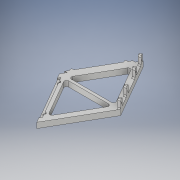
# Autodesk Inventor part: Hex_Servo_Base
Saved by Autodesk Inventor 2019 (Build 230136000, 136)
## iProperties
Created: 2019-09-23
Part Number: Hex_Servo_Base
Material: Generic
Document SubType Name: Modeling
Designer: Jorian Brusind
Density: 1 g/cm^3
Appearance: Default
Author: Jorian Brusind
Autodesk Inventor part; units mm, degrees
ref_plane "YZ Plane" through (0, 0, 0) normal (1, 0, 0) x (0, 1, 0)
ref_plane "XZ Plane" through (0, 0, 0) normal (0, 1, 0) x (-1, 0, 0)
ref_plane "XY Plane" through (0, 0, 0) normal (0, 0, 1) x (1, 0, 0)
sketch "Sketch5" plane through (0, 0, 0) normal (0, 1, 0) x (-1, 0, 0)
  line L0 (0, 0) -> (-90, 0)
  line L1 (-90, 0) -> (-45, 77.9423)
  line L2 (-90, 0) -> (-45, -77.9423)
  line L3 (-90, 0) -> (0, 0) construction
  line L4 (-45, 77.9423) -> (0, 0)
  line L5 (-45, -77.9423) -> (0, 0)
  line L6 (11.547, 0) -> (-45, 97.9423)
  line L7 (-45, 97.9423) -> (-101.547, 0)
  line L8 (-101.547, 0) -> (-45, -97.9423)
  line L9 (-45, -97.9423) -> (11.547, 0)
  line L10 (-90, -2.5) -> (0, -2.5)
  line L11 (0, -2.5) -> (0, 2.5)
  line L12 (0, 2.5) -> (-90, 2.5)
  line L13 (-90, 2.5) -> (-90, -2.5)
  line L14 (-90, -2.5) -> (0, 2.5) construction
  line L15 (0, -2.5) -> (-90, 2.5) construction
  point P0 (-45, 0)
  dimension "d32" = 90
  dimension "d33" = 90
  dimension "d34" = 60
  dimension "d35" = 90
  dimension "d36" = 60
  dimension "d37" = 60
  dimension "d38" = 10
  dimension "d39" = 5
  constraints: 32 end point, 3 midpoint, 3 parallel, 2 horizontal, 1 equal length, 1 perpendicular, 3 other
  measures "d32" distance of L0.start L0.end
  measures "d33" distance of L0.end L1.end
  measures "d34" angle of L0 L1
  measures "d35" distance of L0.end L2.end
  measures "d36" angle of L2 L3
  measures "d37" angle of L2 L5
  measures "d38" distance between parallel lines of L4 L6
  measures "d39" distance of L11.end L10.end
extrude "Extrusion4" add sketch "Sketch5" along normal blind 10 contours L5 L10 L2 L0 | L0 L1 L12 L4 | L11 L10 L5 | L4 L12 L11 | L13 L12 L1 | L2 L10 L13 | L9 L8 L7 L6
sketch "Sketch6" plane through (0, 10, 0) normal (0, 1, 0) x (1, 0, 0)
  line L0 (-11.547, 0) -> (45, -97.9423) projected
  line L1 (45, -97.9423) -> (40, -89.282)
  line L2 (40, -89.282) -> (42.5, -84.9519)
  line L3 (40, -89.282) -> (45, -89.282) construction
  line L4 (-11.547, 0) -> (-6.547, -8.6603)
  line L5 (-6.547, -8.6603) -> (-4.047, -4.3301)
  line L6 (-6.547, -8.6603) -> (-1.547, -8.6603) construction
  line L7 (-4.047, -4.3301) -> (42.5, -84.9519)
  line L8 (40, -89.282) -> (-6.547, -8.6603)
  point P0 (0, 0)
  dimension "d42" = 10
  dimension "d43" = 5
  dimension "d44" = 60
  dimension "d45" = 10
  dimension "d46" = 5
  dimension "d47" = 60
  constraints: 16 end point, 2 equal length, 2 horizontal, 2 point on line, 1 collinear
  measures "d42" distance of L0.end L1.end
  measures "d43" distance of L1.end L2.end
  measures "d44" angle of L3 L2
  measures "d45" distance of L0.start L4.end
  measures "d46" distance of L4.end L5.end
  measures "d47" angle of L6 L5
extrude "Extrusion5" cut sketch "Sketch6" against normal blind 3
sketch "Sketch7" plane through (0, 10, 0) normal (0, 1, 0) x (1, 0, 0)
  line L0 (-4.047, -4.3301) -> (0.953, -12.9904)
  line L1 (-4.047, -4.3301) -> (42.5, -84.9519) projected
  circle A0 centre (0.953, -12.9904) radius 2.5
  line L2 (42.5, -84.9519) -> (37.5, -76.2917)
  line L3 (42.5, -84.9519) -> (52.5, -84.9519) construction
  circle A1 centre (37.5, -76.2917) radius 2.5
  point P0 (0, 0)
  dimension "d50" = 10
  dimension "d51" = 5
  dimension "d52" = 10
  dimension "d53" = 120
  dimension "d54" = 5
  constraints: 6 end point, 2 centre point, 2 coincident, 1 collinear, 1 equal length, 1 horizontal, 1 point on line
  measures "d50" distance of L0.start L0.end
  measures "d51" diameter of A0
  measures "d52" distance of L1.end L2.end
  measures "d53" angle of L3 L2
  measures "d54" diameter of A1
extrude "Extrusion6" cut sketch "Sketch7" against normal blind 6
sketch "Sketch8" plane through (0, 10, 0) normal (0, 1, 0) x (1, 0, 0)
  line L0 (-11.547, 0) -> (-6.547, -8.6603) projected
  line L1 (-5.4845, 10.5006) -> (-1.547, 10.5006) construction
  line L2 (-5.4845, 10.5006) -> (-0.9845, 10.5006) construction
  line L3 (40, 89.282) -> (44.5, 89.282) construction
  line L4 (-11.547, 0) -> (-6.297, 9.0933)
  line L5 (45, 97.9423) -> (-11.547, 0) projected
  line L6 (-11.547, 0) -> (-1.047, 0) construction
  line L7 (45, 97.9423) -> (39.75, 88.849)
  line L8 (39.75, 88.849) -> (-6.297, 9.0933)
  line L9 (39.75, 88.849) -> (35.25, 88.849)
  line L10 (-6.297, 9.0933) -> (-10.797, 9.0933)
  line L11 (-10.797, 9.0933) -> (35.25, 88.849)
  point P0 (0, 0)
  dimension "d189" = 10.5
  dimension "d190" = 60
  dimension "d191" = 10.5
  dimension "d192" = 4.5
  dimension "d193" = 4.5
  constraints: 20 end point, 6 horizontal, 1 collinear, 1 equal length, 1 point on line
  measures "d189" distance of L0.start L4.end
  measures "d190" angle of L6 L4
  measures "d191" distance of L5.start L7.end
  measures "d192" distance of L7.end L9.end
  measures "d193" distance of L4.end L10.end
sketch "Sketch10" plane through (0, 10, 0) normal (0, 1, 0) x (1, 0, 0)
  line L0 (101.547, 0) -> (45, 97.9423) projected
  line L1 (101.547, 0) -> (99.047, 4.3301)
  line L2 (99.047, 4.3301) -> (85.447, 27.886)
  line L3 (85.447, 27.886) -> (82.947, 32.2161)
  line L4 (82.947, 32.2161) -> (79.4829, 30.2161)
  line L5 (45, 77.9423) -> (88.5566, 2.5) projected
  line L6 (98.5395, -1.7321) -> (105.9395, -1.7321) construction
  line L7 (79.4829, 30.2161) -> (82.9829, 24.154)
  line L8 (82.9829, 24.154) -> (86.447, 26.154)
  line L9 (101.547, 0) -> (98.0829, -2)
  line L10 (101.547, 0) -> (105.547, 0) construction
  line L11 (98.0829, -2) -> (94.5829, 4.0622)
  line L12 (94.5829, 4.0622) -> (98.047, 6.0622)
  line L13 (85.447, 27.886) -> (65.447, 62.527)
  line L14 (101.547, 0) -> (45, 97.9423) projected
  line L15 (65.447, 62.527) -> (62.947, 66.8572)
  line L16 (62.947, 66.8572) -> (49.347, 90.4131)
  line L17 (49.347, 90.4131) -> (46.847, 94.7432)
  line L18 (65.447, 62.527) -> (61.9829, 60.527)
  line L19 (61.9829, 60.527) -> (58.4829, 66.5892)
  line L20 (58.4829, 66.5892) -> (61.947, 68.5892)
  line L21 (46.847, 94.7432) -> (43.3829, 92.7432)
  line L22 (46.847, 94.7432) -> (50.847, 94.7432) construction
  line L23 (43.3829, 92.7432) -> (46.8829, 86.681)
  line L24 (43.3829, 92.7432) -> (50.3829, 92.7432) construction
  line L25 (46.8829, 86.681) -> (50.347, 88.681)
  point P0 (0, 0)
  dimension "d77" = 5
  dimension "d78" = 27.2
  dimension "d83" = 5
  dimension "d84" = 4
  dimension "d93" = 7
  dimension "d94" = 3.4641
  dimension "d101" = 4
  dimension "d102" = 150
  dimension "d103" = 7
  dimension "d104" = 90
  dimension "d107" = 40
  dimension "d108" = 5
  dimension "d109" = 27.2
  dimension "d110" = 5
  dimension "d111" = 4
  dimension "d112" = 7
  dimension "d113" = 4
  dimension "d114" = 150
  dimension "d115" = 7
  dimension "d116" = 60
  constraints: 46 end point, 8 perpendicular, 8 point on line, 4 horizontal, 3 equal length, 4 other
  measures "d77" distance of L0.start L1.end
  measures "d78" distance of L1.end L2.end
  measures "d83" distance of L2.end L3.end
  measures "d84" distance of L3.end L4.end
  measures "d93" distance of L4.end L7.end
  measures "d94" horizontal distance of L7.end L8.end
  measures "d101" distance of L0.start L9.end
  measures "d102" angle of L9 L10
  measures "d103" distance of L9.end L11.end
  measures "d104" angle of L9 L11
  measures "d107" distance of L2.end L13.end
  measures "d108" distance of L13.end L15.end
  measures "d109" distance of L15.end L16.end
  measures "d110" distance of L16.end L17.end
  measures "d111" distance of L13.end L18.end
  measures "d112" distance of L18.end L19.end
  measures "d113" distance of L17.end L21.end
  measures "d114" angle of L21 L22
  measures "d115" distance of L21.end L23.end
  measures "d116" angle of L23 L24
extrude "Extrusion10" add sketch "Sketch10" along normal blind 15
sketch "Sketch11" plane through (45, 0, -97.9423) normal (0.8660254, 0, -0.5) x (-0.5, 0, -0.8660254)
  line L0 (-106.094, 10) -> (-82.894, 10) projected
  line L1 (-106.094, 10) -> (-106.094, 17)
  line L2 (-106.094, 10) -> (-106.094, 25) projected
  line L3 (-106.094, 17) -> (-108.294, 17)
  circle A0 centre (-108.294, 17) radius 1.25
  circle A1 centre (-81.094, 17) radius 1.25
  line L4 (-33.894, 10) -> (-33.894, 25) projected
  line L5 (-33.894, 10) -> (-33.894, 17)
  line L6 (-33.894, 17) -> (-36.094, 17)
  circle A2 centre (-36.094, 17) radius 1.25
  circle A3 centre (-8.894, 17) radius 1.25
  point P0 (-62.3205, 0)
  dimension "d119" = 7
  dimension "d120" = 2.2
  dimension "d121" = 2.5
  dimension "d124" = 27.2
  dimension "d129" = 7
  dimension "d130" = 2.2
  dimension "d131" = 2.5
  dimension "d134" = 27.2
  constraints: 8 end point, 4 centre point, 2 coincident, 2 horizontal, 2 perpendicular, 2 point on line, 4 other
  measures "d119" distance of L0.start L1.end
  measures "d120" distance of L1.end L3.end
  measures "d121" diameter of A0
  measures "d124" distance of A0.centre A1.centre
  measures "d129" distance of L4.start L5.end
  measures "d130" distance of L5.end L6.end
  measures "d131" diameter of A2
  measures "d134" distance of A2.centre A3.centre
extrude "Extrusion11" cut sketch "Sketch11" against normal blind 4
fillet "Fillet3" radius 2 16 edges at (48.615, 10, -87.681) (63.715, 10, -61.527) (84.715, 10, -25.154) (99.815, 10, 1) (96.315, 10, -5.0622) (81.215, 10, -31.2161) (60.215, 10, -67.5892) (45.115, 10, -93.7432) (45.115, 25, -93.7432) (48.615, 25, -87.681) (60.215, 25, -67.5892) (63.715, 25, -61.527) (81.215, 25, -31.2161) (84.715, 25, -25.154) (96.315, 25, -5.0622) (99.815, 25, 1)
fillet "Fillet5" radius 2 4 edges at (38.75, 8.5, 78.4567) (36.25, 8.5, 74.1266) (2.203, 8.5, 15.1554) (-0.297, 8.5, 10.8253)
extrude "Extrusion15" add sketch "Sketch8" against normal blind 3
sketch "Sketch14" plane through (0, 10, 0) normal (0, 1, 0) x (1, 0, 0)
  line L0 (35.25, 88.849) -> (-10.797, 9.0933) projected
  line L1 (35.25, 88.849) -> (30.5, 80.6218)
  line L2 (-10.797, 9.0933) -> (-6.047, 17.3205)
  line L3 (-6.047, 17.3205) -> (-6.48, 17.5705)
  line L4 (-6.047, 17.3205) -> (-5.547, 17.3205) construction
  line L5 (30.5, 80.6218) -> (30.067, 80.8718)
  line L6 (30.5, 80.6218) -> (31, 80.6218) construction
  circle A0 centre (30.067, 80.8718) radius 2.3
  circle A1 centre (-6.48, 17.5705) radius 2.3
  point P0 (0, 0)
  dimension "d196" = 9.5
  dimension "d197" = 9.5
  dimension "d198" = 0.5
  dimension "d199" = 150
  dimension "d200" = 0.5
  dimension "d201" = 150
  dimension "d202" = 4.6
  dimension "d203" = 4.6
  constraints: 12 end point, 2 centre point, 2 coincident, 2 equal length, 2 horizontal, 2 point on line, 1 perpendicular
  measures "d196" distance of L0.start L1.end
  measures "d197" distance of L0.end L2.end
  measures "d198" distance of L2.end L3.end
  measures "d199" angle of L4 L3
  measures "d200" distance of L1.end L5.end
  measures "d201" angle of L6 L5
  measures "d202" diameter of A0
  measures "d203" diameter of A1
extrude "Extrusion16" add sketch "Sketch14" against normal blind 6
fillet "Fillet8" radius 4 6 edges at (1.4434, 5, 2.5) (1.4434, 5, -2.5) (88.5566, 5, 2.5) (88.5566, 5, -2.5) (45, 5, 77.9423) (45, 5, -77.9423)
fillet "Fillet9" radius 2 4 edges at (-7.1695, 8.5, -15.3763) (-4.9245, 8.5, -19.2647) (31.6225, 8.5, -82.566) (29.3775, 8.5, -78.6776)
body "Solid2"
